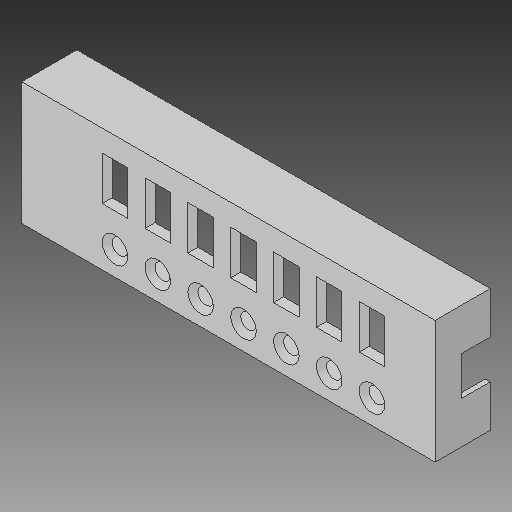
# Autodesk Inventor part: cover
Saved by Autodesk Inventor 2019 (Build 230136000, 136)
## iProperties
Created: 2019-04-16
Part Number: cover
Material: Generic
Document SubType Name: Modeling
Designer: zacha
Density: 1 g/cm^3
Appearance: Default
Author: zacha
Autodesk Inventor part; units mm, degrees
ref_plane "YZ Plane" through (0, 0, 0) normal (1, 0, 0) x (0, 1, 0)
ref_plane "XZ Plane" through (0, 0, 0) normal (0, 1, 0) x (-1, 0, 0)
ref_plane "XY Plane" through (0, 0, 0) normal (0, 0, 1) x (1, 0, 0)
sketch "Sketch1" plane through (0, 0, 0) normal (0, 0, 1) x (1, 0, 0)
  line L0 (82.5, -24.5) -> (-82.5, -24.5)
  line L1 (-82.5, -24.5) -> (-82.5, 24.5)
  line L2 (-82.5, 24.5) -> (82.5, 24.5)
  line L3 (82.5, 24.5) -> (82.5, -24.5)
  circle A0 centre (-28.2, -14.95) radius 3.1 projected
  circle A1 centre (6, -14.95) radius 3.1 projected
  circle A2 centre (40.2, -14.95) radius 3.1 projected
  circle A3 centre (57.3, -14.95) radius 3.1 projected
  circle A4 centre (23.1, -14.95) radius 3.1 projected
  circle A5 centre (-11.1, -14.95) radius 3.1 projected
  circle A6 centre (-45.3, -14.95) radius 3.1 projected
  line L4 (-25.1, 0.4) -> (-31.3, 0.4) projected
  line L5 (-31.3, 0.4) -> (-31.3, 13.9) projected
  line L6 (-31.3, 13.9) -> (-25.1, 13.9) projected
  line L7 (-25.1, 13.9) -> (-25.1, 0.4) projected
  line L8 (9.1, 0.4) -> (2.9, 0.4) projected
  line L9 (2.9, 0.4) -> (2.9, 13.9) projected
  line L10 (2.9, 13.9) -> (9.1, 13.9) projected
  line L11 (9.1, 13.9) -> (9.1, 0.4) projected
  line L12 (43.3, 0.4) -> (37.1, 0.4) projected
  line L13 (37.1, 0.4) -> (37.1, 13.9) projected
  line L14 (37.1, 13.9) -> (43.3, 13.9) projected
  line L15 (43.3, 13.9) -> (43.3, 0.4) projected
  line L16 (54.2, 0.4) -> (54.2, 13.9) projected
  line L17 (54.2, 13.9) -> (60.4, 13.9) projected
  line L18 (60.4, 13.9) -> (60.4, 0.4) projected
  line L19 (60.4, 0.4) -> (54.2, 0.4) projected
  line L20 (26.2, 0.4) -> (20, 0.4) projected
  line L21 (20, 0.4) -> (20, 13.9) projected
  line L22 (20, 13.9) -> (26.2, 13.9) projected
  line L23 (26.2, 13.9) -> (26.2, 0.4) projected
  line L24 (-8, 0.4) -> (-14.2, 0.4) projected
  line L25 (-14.2, 0.4) -> (-14.2, 13.9) projected
  line L26 (-14.2, 13.9) -> (-8, 13.9) projected
  line L27 (-8, 13.9) -> (-8, 0.4) projected
  line L28 (-42.2, 0.4) -> (-48.4, 0.4) projected
  line L29 (-48.4, 0.4) -> (-48.4, 13.9) projected
  line L30 (-48.4, 13.9) -> (-42.2, 13.9) projected
  line L31 (-42.2, 13.9) -> (-42.2, 0.4) projected
  arc A7 (73.05, -22.25) -> (80.25, -15.05) centre (73.05, -15.05) ccw projected
  line L32 (80.25, -15.05) -> (80.25, 15.05) projected
  arc A8 (80.25, 15.05) -> (73.05, 22.25) centre (73.05, 15.05) ccw projected
  line L33 (73.05, 22.25) -> (-73.05, 22.25) projected
  arc A9 (-73.05, 22.25) -> (-80.25, 15.05) centre (-73.05, 15.05) ccw projected
  line L34 (-80.25, 15.05) -> (-80.25, -15.05) projected
  arc A10 (-80.25, -15.05) -> (-73.05, -22.25) centre (-73.05, -15.05) ccw projected
  line L35 (-73.05, -22.25) -> (73.05, -22.25) projected
  line L36 (-73.05, -22.25) -> (73.05, -22.25) projected
  point P0 (0, 0)
  dimension "d0" = 2.25
  dimension "d1" = 2.25
  dimension "d2" = 2.25
  dimension "d3" = 2.25
  constraints: 8 end point, 2 parallel, 1 horizontal, 1 perpendicular
  measures "d0" distance between parallel lines of L35 L0
  measures "d1" distance between parallel lines of L34 L1
  measures "d2" distance between parallel lines of L33 L2
  measures "d3" distance between parallel lines of L3 L32
extrude "Extrusion1" add sketch "Sketch1" along normal blind 2 contours L0 L1 L2 L3 | L35 A10 L34 A9 L33 A8 L32 A7
sketch "Sketch2" plane through (0, 0, 0) normal (0, 0, -1) x (-1, 0, 0)
  line L0 (-82.5, -24.5) -> (-82.5, 24.5) projected
  line L1 (-82.5, -24.5) -> (-80.5, -24.5)
  line L2 (-80.5, -24.5) -> (-80.5, 24.5)
  line L3 (-80.5, 24.5) -> (-82.5, 24.5)
  line L4 (-82.5, 24.5) -> (-82.5, -24.5)
  line L5 (82.5, 24.5) -> (-82.5, 24.5) projected
  line L6 (82.5, 24.5) -> (82.5, -24.5) projected
  line L7 (-82.5, -24.5) -> (82.5, -24.5)
  line L8 (82.5, -24.5) -> (82.5, -22.5)
  line L9 (82.5, -22.5) -> (-82.5, -22.5)
  line L10 (-82.5, -22.5) -> (-82.5, -24.5)
  line L11 (82.5, -24.5) -> (-82.5, -24.5) projected
  line L12 (-82.5, 24.5) -> (82.5, 24.5) projected
  line L13 (82.5, -24.5) -> (80.5, -24.5)
  line L14 (80.5, -24.5) -> (80.5, 24.5)
  line L15 (80.5, 24.5) -> (82.5, 24.5)
  line L16 (82.5, 24.5) -> (82.5, -24.5)
  line L17 (82.5, 24.5) -> (-82.5, 24.5)
  line L18 (-82.5, 24.5) -> (-82.5, 22.5)
  line L19 (-82.5, 22.5) -> (82.5, 22.5)
  line L20 (82.5, 22.5) -> (82.5, 24.5)
  point P0 (0, 0)
  dimension "d6" = 2
  dimension "d7" = 2
  dimension "d8" = 2
  dimension "d9" = 2
  constraints: 32 end point, 8 parallel, 4 horizontal, 4 perpendicular, 3 point on line, 2 collinear
  measures "d6" distance of L3.end L2.end
  measures "d7" distance of L8.end L7.end
  measures "d8" distance of L14.end L15.end
  measures "d9" distance of L18.end L17.end
extrude "Extrusion2" add sketch "Sketch2" along normal blind 20 contours L0 L9 L2 L1 | L0 L19 L2 L9 | L2 L9 L14 L7 | L0 L3 L2 L19 | L14 L9 L6 L7 | L2 L5 L14 L19 | L14 L19 L6 L9 | L14 L5 L6 L19
sketch "Sketch3" plane through (-82.5, -24.5, 2) normal (-1, 0, 0) x (0, 0, 1)
  circle A0 centre (-15.3, 16.55) radius 5.3 construction
  circle A1 centre (-16.35, 35.4) radius 2.25 construction
  arc A2 (-16.35, 32.15) -> (-16.35, 38.65) centre (-16.35, 35.4) ccw
  arc A3 (-15.3, 10.25) -> (-15.3, 22.85) centre (-15.3, 16.55) ccw
  line L0 (-16.35, 38.65) -> (-22, 38.65)
  line L1 (-22, 2) -> (-22, 47) projected
  line L2 (-16.35, 32.15) -> (-22, 32.15)
  line L3 (-15.3, 22.85) -> (-22, 22.85)
  line L4 (-15.3, 10.25) -> (-22, 10.25)
  line L5 (-22, 10.25) -> (-22, 22.85)
  line L6 (-22, 32.15) -> (-22, 38.65)
  arc A4 (-15.3, 22.85) -> (-15.3, 10.25) centre (-15.3, 16.55) ccw construction
  arc A5 (-16.35, 38.65) -> (-16.35, 32.15) centre (-16.35, 35.4) ccw construction
  point P0 (-2, 24.5)
  dimension "d12" = 1
  dimension "d13" = 1
  constraints: 12 end point, 8 point on circle, 4 centre point, 4 tangent, 3 point on line, 2 coincident, 2 collinear, 2 horizontal, 1 parallel, 1 perpendicular
  measures "d12" radial gap between concentric circles of A1 A2
  measures "d13" radial gap between concentric circles of A3 A0
extrude "Extrusion3" cut sketch "Sketch3" against normal blind 20
sketch "Sketch4" plane through (82.5, -24.5, 2) normal (1, 0, 0) x (0, 0, -1)
  line L0 (18.25, 17.75) -> (11.45, 17.75) projected
  line L1 (11.45, 17.75) -> (11.45, 31.25) projected
  line L2 (11.45, 31.25) -> (18.25, 31.25) projected
  line L3 (18.25, 31.25) -> (18.25, 17.75) projected
  line L4 (25.6, 9.45) -> (2, 9.45) projected
  line L5 (25.6, 39.55) -> (25.6, 9.45) projected
  line L6 (2, 39.55) -> (25.6, 39.55) projected
  line L7 (2, 9.45) -> (2, 39.55) projected
  line L8 (10.45, 16.75) -> (22, 16.75)
  line L9 (22, 16.75) -> (22, 32.25)
  line L10 (22, 32.25) -> (10.45, 32.25)
  line L11 (10.45, 32.25) -> (10.45, 16.75)
  line L12 (22, 49) -> (22, 0) projected
  point P0 (2, 24.5)
  dimension "d16" = 1
  dimension "d17" = 1
  dimension "d19" = 1
  constraints: 8 end point, 2 parallel, 1 collinear, 1 horizontal, 1 perpendicular
  measures "d16" distance between parallel lines of L0 L8
  measures "d17" distance between parallel lines of L2 L10
  measures "d19" distance between parallel lines of L1 L11
extrude "Extrusion4" cut sketch "Sketch4" against normal blind 20 contours L0 L1 L2 L3 | L8 L11 L10 L9
chamfer "Chamfer1" distance 2 angle 45 35 edges at (-45.3, 13.9, 2) (-48.4, 7.15, 2) (-45.3, 0.4, 2) (-42.2, 7.15, 2) (-31.3, 7.15, 2) (-28.2, 13.9, 2) (-25.1, 7.15, 2) (-28.2, 0.4, 2) (-14.2, 7.15, 2) (-11.1, 13.9, 2) (-8, 7.15, 2) (-11.1, 0.4, 2) (2.9, 7.15, 2) (6, 13.9, 2) (9.1, 7.15, 2) (6, 0.4, 2) (26.2, 7.15, 2) (23.1, 13.9, 2) (20, 7.15, 2) (23.1, 0.4, 2) (40.2, 0.4, 2) (37.1, 7.15, 2) (40.2, 13.9, 2) (43.3, 7.15, 2) (54.2, 7.15, 2) (57.3, 13.9, 2) (60.4, 7.15, 2) (57.3, 0.4, 2) (54.2, -14.95, 2) (37.1, -14.95, 2) (20, -14.95, 2) (2.9, -14.95, 2) (-14.2, -14.95, 2) (-31.3, -14.95, 2) (-48.4, -14.95, 2)
equation "\"d1\" = d0"
equation "\"d2\" = d0"
equation "\"d3\" = d0"
equation "\"d17\" = d16"
equation "\"d19\" = d16"
body "Solid1"
